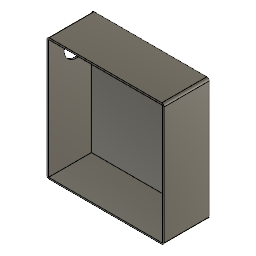
Final Project Box v6 (Autodesk Fusion 360 design; units mm, degrees)
Autodesk Fusion 360 part; units mm, degrees
sketch "Sketch1" plane through (0, 0, 0) normal (0, 1, 0) x (1, 0, 0) in component "Box"
  line L0 (0, 0) -> (80, 0)
  line L1 (80, 0) -> (80, -60)
  line L2 (80, -60) -> (0, -60)
  line L3 (0, -60) -> (0, 0)
  dimension "d1" = 60
  dimension "d2" = 80
  constraint horizontal L0
  constraint vertical L1
  constraint horizontal L2
  constraint vertical L3
  constraint coincident L0.start L3.end
  measures "d1" distance of L0.start L2.end
  measures "d2" distance of L0.start L0.end
extrude "Extrude1" add sketch "Sketch1" along normal blind 47.5 in component "Box"
sketch "Sketch2" plane through (0, 0, 0) normal (0, 1, 0) x (1, 0, 0) in component "Box"
  line L0 (75, -5) -> (5, -5)
  line L1 (5, -5) -> (5, -55)
  line L2 (5, -55) -> (75, -55)
  line L3 (75, -55) -> (75, -5)
  line L4 (75, -5) -> (5, -55) construction
  line L5 (5, -5) -> (75, -55) construction
  line L6 (0, 0) -> (0, -60)
  point P0 (40, -30)
  point P1 (80, 0)
  point P2 (80, -60)
  dimension "d5" = 70
  dimension "d6" = 50
  dimension "d7" = 60
  dimension "d8" = 60
  constraint perpendicular L0 L1
  constraint parallel L0 L2
  constraint parallel L1 L3
  constraint horizontal L0
  constraint coincident L4 P0
  constraint coincident L5 P0
  measures "d5" distance of L1.end L2.end
  measures "d6" distance of L0.end L1.end
  measures "d7" distance of P1 P2
  measures "d8" distance of L6.start L6.end
extrude "Extrude2" cut sketch "Sketch2" along normal blind 45 in component "Box"
fillet "Fillet1" radius 2.5 2 edges at (0, 23.75, 60) (0, 23.75, 0) in component "Box"
fillet "Fillet2" radius 2.5 2 edges at (80, 23.75, 60) (80, 23.75, 0) in component "Box"
sketch "Sketch3" plane through (0, 0, 0) normal (-1, 0, 0) x (0, -1, 0) in component "Box"
  line L0 (-47.5, 2.5) -> (0, 2.5)
  line L1 (0, 2.5) -> (0, 57.5)
  line L2 (0, 57.5) -> (-47.5, 57.5)
  line L3 (-47.5, 57.5) -> (-47.5, 2.5)
  circle A0 centre (-30, 40) radius 13.335
  dimension "d13" = 26.67
  measures "d13" diameter of A0
extrude "Extrude3" cut sketch "Sketch3" against normal blind 30 contours A0 in component "Box"
delete_face "DeleteFace1" 1 faces at (1.6667, 16.7313, 38.6723) in component "Box"
sketch "Sketch1 (2)" plane through (0, 0, 0) normal (-1, 0, 0) x (0, -1, 0)
  line L0 (-47.5, 2.5) -> (0, 2.5)
  line L1 (0, 2.5) -> (0, 57.5)
  line L2 (0, 57.5) -> (-47.5, 57.5)
  line L3 (-47.5, 57.5) -> (-47.5, 2.5)
  circle A0 centre (-30, 40) radius 13.5
  dimension "d16" = 27
  measures "d16" diameter of A0
extrude "Extrude4" cut sketch "Sketch1 (2)" against normal blind 50 contours A0 in component "Box"
delete_face "DeleteFace2" 1 faces at (78.4292, 15.8333, 0.1791) in component "Box"
delete_face "DeleteFace3" 1 faces at (77.9731, 15.8333, 59.9548) in component "Box"
extrude "Extrude5" add 1 faces at (80, 15.8333, 20) along direction (1, 0, 0) blind 43.18 in component "Box"
extrude "Extrude6" cut 1 faces at (75, 15, 38.3333) along direction (1, 0, 0) blind 45 in component "Box"
delete_face "DeleteFace4" 1 faces at (0.0028, 15.8333, 2.381) in component "Box"
delete_face "DeleteFace5" 1 faces at (2.381, 15.8333, 59.9972) in component "Box"
extrude "Extrude7" add 1 faces at (41.06, 31.6667, 0) along direction (0, 0, -1) blind 68.58 in component "Box"
extrude "Extrude8" cut 1 faces at (43.3333, 15, 5) along direction (0, 0, -1) blind 70 in component "Box"
extrude "Extrude9" cut 1 faces at (5, 24.6637, -34.4874) along direction (-1, 0, 0) blind 2 in component "Box"
extrude "Extrude10" cut 1 faces at (81, 30, 55) along direction (0, 0, 1) blind 2 in component "Box"
fillet "Fillet3" radius 2.5 1 edges at (123.18, 23.75, -68.58) in component "Box"
fillet "Fillet4" radius 2.5 1 edges at (0, 23.75, -68.58) in component "Box"
fillet "Fillet5" radius 2.5 1 edges at (0, 23.75, 60) in component "Box"
fillet "Fillet6" radius 2.5 1 edges at (123.18, 23.75, 60) in component "Box"
extrude "Extrude11" cut 1 faces at (42, 15, -65) along direction (0, 0, -1) blind 2 in component "Box"
extrude "Extrude12" cut 1 faces at (81, 30, 57) along direction (0, 0, 1) blind 0.15 in component "Box"
extrude "Extrude13" cut 1 faces at (81, 30, 57.15) along direction (0, 0, 1) blind 0.5 in component "Box"
extrude "Extrude14" cut 1 faces at (81, 30, 57.65) along direction (0, 0, 1) blind 0.5 in component "Box"
extrude "Extrude15" cut 1 faces at (120, 15, -25.2833) along direction (1, 0, 0) blind 0.5 in component "Box"
extrude "Extrude16" cut 1 faces at (120.5, 15, -25.2833) along direction (1, 0, 0) blind 0.5 in component "Box"
extrude "Extrude17" cut 1 faces at (121, 15, -25.2833) along direction (1, 0, 0) blind 0.3 in component "Box"
extrude "Extrude18" cut 1 faces at (121.3, 15, -25.2833) along direction (1, 0, 0) blind 0.2 in component "Box"
extrude "Extrude19" cut 1 faces at (3, 24.6637, -35.8208) along direction (-1, 0, 0) blind 2 in component "Box"
extrude "Extrude20" add 1 faces at (1, 24.6637, -35.8208) along direction (1, 0, 0) blind 0.5 in component "Box"
extrude "Extrude21" add 1 faces at (1.5, 24.6637, -35.8208) along direction (1, 0, 0) blind 0.5 in component "Box"
component "Box" placed x (1, 0, 0) y (0, 1, 0) z (0, 0, 1) at (0, 0, 0)
